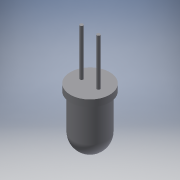
# Autodesk Inventor part: ledka
Saved by Autodesk Inventor 2018 (Build 220112000, 112)
## iProperties
Created: 2019-01-22
Part Number: ledka
Material: Glass
Document SubType Name: Modeling
Designer: petal
Density: 2.18 g/cm^3
Appearance: Clear
Author: petal
Autodesk Inventor part; units mm, degrees
ref_plane "YZ Plane" through (0, 0, 0) normal (1, 0, 0) x (0, 1, 0)
ref_plane "XZ Plane" through (0, 0, 0) normal (0, 1, 0) x (-1, 0, 0)
ref_plane "XY Plane" through (0, 0, 0) normal (0, 0, 1) x (1, 0, 0)
sketch "Sketch1" plane through (0, 0, 0) normal (0, 1, 0) x (-1, 0, 0)
  line L0 (0, 0) -> (0, -8.7)
  line L1 (0, 0) -> (2.95, 0)
  line L2 (2.95, 0) -> (2.95, -1)
  line L3 (2.95, -1) -> (2.5, -1)
  line L4 (2.5, -1) -> (2.5, -6.2)
  arc A0 (0, -8.7) -> (2.5, -6.2) centre (0, -6.2) ccw
  dimension "d0" = 8.7
  dimension "d1" = 5.9
  dimension "d2" = 1
  dimension "d3" = 5
  constraints: 10 end point, 3 perpendicular, 2 point on circle, 1 centre point, 1 horizontal, 1 point on line, 1 tangent, 1 vertical
  measures "d0" distance of L0.start L0.end
  measures "d1" diameter of L2 L0
  measures "d2" distance of L2.end L1.end
  measures "d3" diameter of L4 L0
revolve "Revolution1" add sketch "Sketch1" angle 360 about axis through (0, 0, 0) along (0, 0, -1)
sketch "Sketch2" plane through (0, 0, 0) normal (0, 0, 1) x (1, 0, 0)
  circle A0 centre (-1.27, 0) radius 0.25
  circle A1 centre (1.27, 0) radius 0.25
  point P0 (0, 0)
  dimension "d5" = 2.54
  dimension "d6" = 1.27
  dimension "d7" = 0.5
  dimension "d8" = 0.5
  constraints: 2 centre point
  measures "d5" distance of A1.centre A0.centre
  measures "d6" distance of A0.centre point (0, 0)
  measures "d7" diameter of A0
  measures "d8" diameter of A1
extrude "Extrusion1" add sketch "Sketch2" along normal blind 4
equation "\"d6\" = 0.5 * d5"
body "Solid1"
